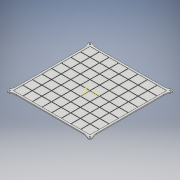
# Autodesk Inventor part: base
Saved by Autodesk Inventor 2017 (Build 210142000, 142)
## iProperties
Created: 2019-02-08
Part Number: base
Material: Generic
Document SubType Name: Modeling
Designer: felix
Density: 1 g/cm^3
Appearance: Default
Author: felix
Autodesk Inventor part; units mm, degrees
ref_plane "YZ Plane" through (0, 0, 0) normal (1, 0, 0) x (0, 1, 0)
ref_plane "XZ Plane" through (0, 0, 0) normal (0, 1, 0) x (-1, 0, 0)
ref_plane "XY Plane" through (0, 0, 0) normal (0, 0, 1) x (1, 0, 0)
sketch "Sketch1" plane through (0, 0, 0) normal (0, 1, 0) x (-1, 0, 0)
  line L0 (0, 0) -> (0, 700)
  line L1 (0, 0) -> (0, -700)
  line L2 (0, 0) -> (700, 0)
  line L3 (0, 0) -> (-700, 0)
  line L4 (-207, 207) -> (-157, 207)
  line L5 (-157, 207) -> (-157, 157)
  line L6 (-157, 157) -> (-207, 157)
  line L7 (-207, 157) -> (-207, 207)
  line L8 (-157, 105) -> (-207, 105)
  line L9 (-157, 155) -> (-157, 105)
  line L10 (-207, 155) -> (-157, 155)
  line L11 (-207, 105) -> (-207, 155)
  line L12 (-157, 53) -> (-207, 53)
  line L13 (-157, 103) -> (-157, 53)
  line L14 (-207, 103) -> (-157, 103)
  line L15 (-207, 53) -> (-207, 103)
  line L16 (-157, 1) -> (-207, 1)
  line L17 (-157, 51) -> (-157, 1)
  line L18 (-207, 51) -> (-157, 51)
  line L19 (-207, 1) -> (-207, 51)
  line L20 (-157, -51) -> (-207, -51)
  line L21 (-157, -1) -> (-157, -51)
  line L22 (-207, -1) -> (-157, -1)
  line L23 (-207, -51) -> (-207, -1)
  line L24 (-157, -103) -> (-207, -103)
  line L25 (-157, -53) -> (-157, -103)
  line L26 (-207, -53) -> (-157, -53)
  line L27 (-207, -103) -> (-207, -53)
  line L28 (-157, -155) -> (-207, -155)
  line L29 (-157, -105) -> (-157, -155)
  line L30 (-207, -105) -> (-157, -105)
  line L31 (-207, -155) -> (-207, -105)
  line L32 (-157, -207) -> (-207, -207)
  line L33 (-157, -157) -> (-157, -207)
  line L34 (-207, -157) -> (-157, -157)
  line L35 (-207, -207) -> (-207, -157)
  line L36 (-105, 157) -> (-155, 157)
  line L37 (-105, 207) -> (-105, 157)
  line L38 (-155, 207) -> (-105, 207)
  line L39 (-155, 157) -> (-155, 207)
  line L40 (-105, 105) -> (-155, 105)
  line L41 (-105, 155) -> (-105, 105)
  line L42 (-155, 155) -> (-105, 155)
  line L43 (-155, 105) -> (-155, 155)
  line L44 (-105, 53) -> (-155, 53)
  line L45 (-105, 103) -> (-105, 53)
  line L46 (-155, 103) -> (-105, 103)
  line L47 (-155, 53) -> (-155, 103)
  line L48 (-105, 1) -> (-155, 1)
  line L49 (-105, 51) -> (-105, 1)
  line L50 (-155, 51) -> (-105, 51)
  line L51 (-155, 1) -> (-155, 51)
  line L52 (-105, -51) -> (-155, -51)
  line L53 (-105, -1) -> (-105, -51)
  line L54 (-155, -1) -> (-105, -1)
  line L55 (-155, -51) -> (-155, -1)
  line L56 (-105, -103) -> (-155, -103)
  line L57 (-105, -53) -> (-105, -103)
  line L58 (-155, -53) -> (-105, -53)
  line L59 (-155, -103) -> (-155, -53)
  line L60 (-105, -155) -> (-155, -155)
  line L61 (-105, -105) -> (-105, -155)
  line L62 (-155, -105) -> (-105, -105)
  line L63 (-155, -155) -> (-155, -105)
  line L64 (-105, -207) -> (-155, -207)
  line L65 (-105, -157) -> (-105, -207)
  line L66 (-155, -157) -> (-105, -157)
  line L67 (-155, -207) -> (-155, -157)
  line L68 (-53, 157) -> (-103, 157)
  line L69 (-53, 207) -> (-53, 157)
  line L70 (-103, 207) -> (-53, 207)
  line L71 (-103, 157) -> (-103, 207)
  line L72 (-53, 105) -> (-103, 105)
  line L73 (-53, 155) -> (-53, 105)
  line L74 (-103, 155) -> (-53, 155)
  line L75 (-103, 105) -> (-103, 155)
  line L76 (-53, 53) -> (-103, 53)
  line L77 (-53, 103) -> (-53, 53)
  line L78 (-103, 103) -> (-53, 103)
  line L79 (-103, 53) -> (-103, 103)
  line L80 (-53, 1) -> (-103, 1)
  line L81 (-53, 51) -> (-53, 1)
  line L82 (-103, 51) -> (-53, 51)
  line L83 (-103, 1) -> (-103, 51)
  line L84 (-53, -51) -> (-103, -51)
  line L85 (-53, -1) -> (-53, -51)
  line L86 (-103, -1) -> (-53, -1)
  line L87 (-103, -51) -> (-103, -1)
  line L88 (-53, -103) -> (-103, -103)
  line L89 (-53, -53) -> (-53, -103)
  line L90 (-103, -53) -> (-53, -53)
  line L91 (-103, -103) -> (-103, -53)
  line L92 (-53, -155) -> (-103, -155)
  line L93 (-53, -105) -> (-53, -155)
  line L94 (-103, -105) -> (-53, -105)
  line L95 (-103, -155) -> (-103, -105)
  line L96 (-53, -207) -> (-103, -207)
  line L97 (-53, -157) -> (-53, -207)
  line L98 (-103, -157) -> (-53, -157)
  line L99 (-103, -207) -> (-103, -157)
  line L100 (-1, 157) -> (-51, 157)
  line L101 (-1, 207) -> (-1, 157)
  line L102 (-51, 207) -> (-1, 207)
  line L103 (-51, 157) -> (-51, 207)
  line L104 (-1, 105) -> (-51, 105)
  line L105 (-1, 155) -> (-1, 105)
  line L106 (-51, 155) -> (-1, 155)
  line L107 (-51, 105) -> (-51, 155)
  line L108 (-1, 53) -> (-51, 53)
  line L109 (-1, 103) -> (-1, 53)
  line L110 (-51, 103) -> (-1, 103)
  line L111 (-51, 53) -> (-51, 103)
  line L112 (-1, 1) -> (-51, 1)
  line L113 (-1, 51) -> (-1, 1)
  line L114 (-51, 51) -> (-1, 51)
  line L115 (-51, 1) -> (-51, 51)
  line L116 (-1, -51) -> (-51, -51)
  line L117 (-1, -1) -> (-1, -51)
  line L118 (-51, -1) -> (-1, -1)
  line L119 (-51, -51) -> (-51, -1)
  line L120 (-1, -103) -> (-51, -103)
  line L121 (-1, -53) -> (-1, -103)
  line L122 (-51, -53) -> (-1, -53)
  line L123 (-51, -103) -> (-51, -53)
  line L124 (-1, -155) -> (-51, -155)
  line L125 (-1, -105) -> (-1, -155)
  line L126 (-51, -105) -> (-1, -105)
  line L127 (-51, -155) -> (-51, -105)
  line L128 (-1, -207) -> (-51, -207)
  line L129 (-1, -157) -> (-1, -207)
  line L130 (-51, -157) -> (-1, -157)
  line L131 (-51, -207) -> (-51, -157)
  line L132 (51, 157) -> (1, 157)
  line L133 (51, 207) -> (51, 157)
  line L134 (1, 207) -> (51, 207)
  line L135 (1, 157) -> (1, 207)
  line L136 (51, 105) -> (1, 105)
  line L137 (51, 155) -> (51, 105)
  line L138 (1, 155) -> (51, 155)
  line L139 (1, 105) -> (1, 155)
  line L140 (51, 53) -> (1, 53)
  line L141 (51, 103) -> (51, 53)
  line L142 (1, 103) -> (51, 103)
  line L143 (1, 53) -> (1, 103)
  line L144 (51, 1) -> (1, 1)
  line L145 (51, 51) -> (51, 1)
  line L146 (1, 51) -> (51, 51)
  line L147 (1, 1) -> (1, 51)
  line L148 (51, -51) -> (1, -51)
  line L149 (51, -1) -> (51, -51)
  line L150 (1, -1) -> (51, -1)
  line L151 (1, -51) -> (1, -1)
  line L152 (51, -103) -> (1, -103)
  line L153 (51, -53) -> (51, -103)
  line L154 (1, -53) -> (51, -53)
  line L155 (1, -103) -> (1, -53)
  line L156 (51, -155) -> (1, -155)
  line L157 (51, -105) -> (51, -155)
  line L158 (1, -105) -> (51, -105)
  line L159 (1, -155) -> (1, -105)
  line L160 (51, -207) -> (1, -207)
  line L161 (51, -157) -> (51, -207)
  line L162 (1, -157) -> (51, -157)
  line L163 (1, -207) -> (1, -157)
  line L164 (103, 157) -> (53, 157)
  line L165 (103, 207) -> (103, 157)
  line L166 (53, 207) -> (103, 207)
  line L167 (53, 157) -> (53, 207)
  line L168 (103, 105) -> (53, 105)
  line L169 (103, 155) -> (103, 105)
  line L170 (53, 155) -> (103, 155)
  line L171 (53, 105) -> (53, 155)
  line L172 (103, 53) -> (53, 53)
  line L173 (103, 103) -> (103, 53)
  line L174 (53, 103) -> (103, 103)
  line L175 (53, 53) -> (53, 103)
  line L176 (103, 1) -> (53, 1)
  line L177 (103, 51) -> (103, 1)
  line L178 (53, 51) -> (103, 51)
  line L179 (53, 1) -> (53, 51)
  line L180 (103, -51) -> (53, -51)
  line L181 (103, -1) -> (103, -51)
  line L182 (53, -1) -> (103, -1)
  line L183 (53, -51) -> (53, -1)
  line L184 (103, -103) -> (53, -103)
  line L185 (103, -53) -> (103, -103)
  line L186 (53, -53) -> (103, -53)
  line L187 (53, -103) -> (53, -53)
  line L188 (103, -155) -> (53, -155)
  line L189 (103, -105) -> (103, -155)
  line L190 (53, -105) -> (103, -105)
  line L191 (53, -155) -> (53, -105)
  line L192 (103, -207) -> (53, -207)
  line L193 (103, -157) -> (103, -207)
  line L194 (53, -157) -> (103, -157)
  line L195 (53, -207) -> (53, -157)
  line L196 (155, 157) -> (105, 157)
  line L197 (155, 207) -> (155, 157)
  line L198 (105, 207) -> (155, 207)
  line L199 (105, 157) -> (105, 207)
  line L200 (155, 105) -> (105, 105)
  line L201 (155, 155) -> (155, 105)
  line L202 (105, 155) -> (155, 155)
  line L203 (105, 105) -> (105, 155)
  line L204 (155, 53) -> (105, 53)
  line L205 (155, 103) -> (155, 53)
  line L206 (105, 103) -> (155, 103)
  line L207 (105, 53) -> (105, 103)
  line L208 (155, 1) -> (105, 1)
  line L209 (155, 51) -> (155, 1)
  line L210 (105, 51) -> (155, 51)
  line L211 (105, 1) -> (105, 51)
  line L212 (155, -51) -> (105, -51)
  line L213 (155, -1) -> (155, -51)
  line L214 (105, -1) -> (155, -1)
  line L215 (105, -51) -> (105, -1)
  line L216 (155, -103) -> (105, -103)
  line L217 (155, -53) -> (155, -103)
  line L218 (105, -53) -> (155, -53)
  line L219 (105, -103) -> (105, -53)
  line L220 (155, -155) -> (105, -155)
  line L221 (155, -105) -> (155, -155)
  line L222 (105, -105) -> (155, -105)
  line L223 (105, -155) -> (105, -105)
  line L224 (155, -207) -> (105, -207)
  line L225 (155, -157) -> (155, -207)
  line L226 (105, -157) -> (155, -157)
  line L227 (105, -207) -> (105, -157)
  line L228 (207, 157) -> (157, 157)
  line L229 (207, 207) -> (207, 157)
  line L230 (157, 207) -> (207, 207)
  line L231 (157, 157) -> (157, 207)
  line L232 (207, 105) -> (157, 105)
  line L233 (207, 155) -> (207, 105)
  line L234 (157, 155) -> (207, 155)
  line L235 (157, 105) -> (157, 155)
  line L236 (207, 53) -> (157, 53)
  line L237 (207, 103) -> (207, 53)
  line L238 (157, 103) -> (207, 103)
  line L239 (157, 53) -> (157, 103)
  line L240 (207, 1) -> (157, 1)
  line L241 (207, 51) -> (207, 1)
  line L242 (157, 51) -> (207, 51)
  line L243 (157, 1) -> (157, 51)
  line L244 (207, -51) -> (157, -51)
  line L245 (207, -1) -> (207, -51)
  line L246 (157, -1) -> (207, -1)
  line L247 (157, -51) -> (157, -1)
  line L248 (207, -103) -> (157, -103)
  line L249 (207, -53) -> (207, -103)
  line L250 (157, -53) -> (207, -53)
  line L251 (157, -103) -> (157, -53)
  line L252 (207, -155) -> (157, -155)
  line L253 (207, -105) -> (207, -155)
  line L254 (157, -105) -> (207, -105)
  line L255 (157, -155) -> (157, -105)
  line L256 (207, -207) -> (157, -207)
  line L257 (207, -157) -> (207, -207)
  line L258 (157, -157) -> (207, -157)
  line L259 (157, -207) -> (157, -157)
  circle A0 centre (-217, 217) radius 4
  arc A1 (-211.8492, 225.5714) -> (-225.5714, 211.8492) centre (-217, 217) ccw
  arc A2 (-211.8492, 225.5714) -> (-180.9445, 217) centre (-180.9445, 277) ccw
  arc A3 (-217, 180.9445) -> (-225.5714, 211.8492) centre (-277, 180.9445) ccw
  circle A4 centre (-217, -217) radius 4
  arc A5 (-225.5714, -211.8492) -> (-217, -180.9445) centre (-277, -180.9445) ccw
  arc A6 (-225.5714, -211.8492) -> (-211.8492, -225.5714) centre (-217, -217) ccw
  arc A7 (-180.9445, -217) -> (-211.8492, -225.5714) centre (-180.9445, -277) ccw
  circle A8 centre (217, -217) radius 4
  arc A9 (211.8492, -225.5714) -> (180.9445, -217) centre (180.9445, -277) ccw
  arc A10 (211.8492, -225.5714) -> (225.5714, -211.8492) centre (217, -217) ccw
  arc A11 (217, -180.9445) -> (225.5714, -211.8492) centre (277, -180.9445) ccw
  circle A12 centre (217, 217) radius 4
  arc A13 (225.5714, 211.8492) -> (217, 180.9445) centre (277, 180.9445) ccw
  arc A14 (225.5714, 211.8492) -> (211.8492, 225.5714) centre (217, 217) ccw
  arc A15 (180.9445, 217) -> (211.8492, 225.5714) centre (180.9445, 277) ccw
  line L260 (-217, -180.9445) -> (-217, 180.9445)
  line L261 (180.9445, -217) -> (-180.9445, -217)
  line L262 (217, 180.9445) -> (217, -180.9445)
  line L263 (-180.9445, 217) -> (180.9445, 217)
  dimension "d4" = 50
  dimension "d5" = 50
  dimension "d8" = 52
  dimension "d11" = 52
  dimension "d14" = 700
  dimension "d15" = 2
  dimension "d16" = 2
  dimension "d21" = 8
  dimension "d22" = 20
  dimension "d23" = 60
  dimension "d24" = 60
  dimension "d28" = 360
  dimension "d30" = 60
  dimension "d31" = 543
  dimension "d32" = 857
  dimension "d33" = 917
  constraints: 528 end point, 24 point on circle, 16 centre point, 6 tangent, 5 horizontal, 4 coincident, 4 parallel, 3 vertical, 2 collinear, 2 perpendicular, 551 other
  measures "d4" distance of L5.end L6.end
  measures "d5" distance of L4.end L5.end
  measures "d8" distance of L5.end L8.start
  measures "d11" distance of L5.end L36.start
  measures "d14" distance of L0.start L2.end
  measures "d15" diameter of L16 L2
  measures "d16" diameter of L147 L0
  measures "d21" diameter of A0
  measures "d22" diameter of A1
  measures "d23" radius of A2
  measures "d24" radius of A3
  measures "d30" distance between parallel lines of L228 L263
  measures "d31" distance from line of L0.end L228
  measures "d32" distance from line of L1.end L228
  measures "d33" distance from line of L3.end L262
extrude "Extrusion1" add sketch "Sketch1" against normal blind 5 contours L3 L260 A3 A1 A2 L263 L0 | L2 L262 A11 A10 A9 L261 L1 | L0 L263 A15 A14 A13 L262 L2 | L1 L261 A7 A6 A5 L260 L3 | L4 L5 L6 L7 | L8 L11 L10 L9 | L12 L15 L14 L13 | L16 L19 L18 L17 | L20 L23 L22 L21 | L24 L27 L26 L25 | L28 L31 L30 L29 | L32 L35 L34 L33 | L36 L39 L38 L37 | L40 L43 L42 L41 | L44 L47 L46 L45 | L48 L51 L50 L49 | L52 L55 L54 L53 | L56 L59 L58 L57 | L60 L63 L62 L61 | L64 L67 L66 L65 | L68 L71 L70 L69 | L72 L75 L74 L73 | L76 L79 L78 L77 | L80 L83 L82 L81 | L84 L87 L86 L85 | L88 L91 L90 L89 | L92 L95 L94 L93 | L96 L99 L98 L97 | L100 L103 L102 L101 | L104 L107 L106 L105 | L108 L111 L110 L109 | L112 L115 L114 L113 | L116 L119 L118 L117 | L120 L123 L122 L121 | L124 L127 L126 L125 | L128 L131 L130 L129 | L132 L135 L134 L133 | L136 L139 L138 L137 | L140 L143 L142 L141 | L144 L147 L146 L145 | L148 L151 L150 L149 | L152 L155 L154 L153 | L156 L159 L158 L157 | L160 L163 L162 L161 | L164 L167 L166 L165 | L168 L171 L170 L169 | L172 L175 L174 L173 | L176 L179 L178 L177 | L180 L183 L182 L181 | L184 L187 L186 L185 | L188 L191 L190 L189 | L192 L195 L194 L193 | L196 L199 L198 L197 | L200 L203 L202 L201 | L204 L207 L206 L205 | L208 L211 L210 L209 | L212 L215 L214 L213 | L216 L219 L218 L217 | L220 L223 L222 L221 | L224 L227 L226 L225 | L228 L231 L230 L229 | L232 L235 L234 L233 | L236 L239 L238 L237 | L240 L243 L242 L241 | L244 L247 L246 L245 | L248 L251 L250 L249 | L252 L255 L254 L253 | L256 L259 L258 L257
extrude "Extrusion2" cut sketch "Sketch1" against normal blind 1 contours L4 L5 L6 L7 | L8 L11 L10 L9 | L12 L15 L14 L13 | L16 L19 L18 L17 | L20 L23 L22 L21 | L24 L27 L26 L25 | L28 L31 L30 L29 | L32 L35 L34 L33 | L36 L39 L38 L37 | L40 L43 L42 L41 | L44 L47 L46 L45 | L48 L51 L50 L49 | L52 L55 L54 L53 | L56 L59 L58 L57 | L60 L63 L62 L61 | L64 L67 L66 L65 | L68 L71 L70 L69 | L72 L75 L74 L73 | L76 L79 L78 L77 | L80 L83 L82 L81 | L84 L87 L86 L85 | L88 L91 L90 L89 | L92 L95 L94 L93 | L96 L99 L98 L97 | L100 L103 L102 L101 | L104 L107 L106 L105 | L108 L111 L110 L109 | L112 L115 L114 L113 | L116 L119 L118 L117 | L120 L123 L122 L121 | L124 L127 L126 L125 | L128 L131 L130 L129 | L132 L135 L134 L133 | L136 L139 L138 L137 | L140 L143 L142 L141 | L144 L147 L146 L145 | L148 L151 L150 L149 | L152 L155 L154 L153 | L156 L159 L158 L157 | L160 L163 L162 L161 | L164 L167 L166 L165 | L168 L171 L170 L169 | L172 L175 L174 L173 | L176 L179 L178 L177 | L180 L183 L182 L181 | L184 L187 L186 L185 | L188 L191 L190 L189 | L192 L195 L194 L193 | L196 L199 L198 L197 | L200 L203 L202 L201 | L204 L207 L206 L205 | L208 L211 L210 L209 | L212 L215 L214 L213 | L216 L219 L218 L217 | L220 L223 L222 L221 | L224 L227 L226 L225 | L228 L231 L230 L229 | L232 L235 L234 L233 | L236 L239 L238 L237 | L240 L243 L242 L241 | L244 L247 L246 L245 | L248 L251 L250 L249 | L252 L255 L254 L253 | L256 L259 L258 L257
move or copy body "Move Body1" bodies to move or copy 1 copy no rotation origin (0, 0, 0) rotation axis (1, 0, 0) rotation angle 90 translate (20, 1, 1)
sketch "Sketch2" plane through (-160.9445, 218, 1) normal (0, 0, 1) x (1, 0, 0)
  line L0 (179.9445, -218) -> (179.9445, -268) projected
  line L1 (231.9445, -216) -> (181.9445, -216) projected
  line L2 (179.9445, -218) -> (181.9445, -218)
  line L3 (181.9445, -218) -> (181.9445, -216)
  line L4 (181.9445, -216) -> (179.9445, -216)
  line L5 (179.9445, -216) -> (179.9445, -218)
  point P0 (160.9445, -218)
  point P1 (180.9445, -217)
  constraints: 8 end point, 2 parallel, 1 horizontal, 1 perpendicular
body "Solid1"
